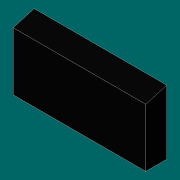
# Autodesk Inventor part: mirrorSuppourt
Saved by Autodesk Inventor 2016 (Build 200138000, 138)
## iProperties
Created: 2015-10-14
Part Number: mirrorSuppourt
Material: PC/ABS Plastic
Document SubType Name: Modeling
Designer: Sawaiz
Density: 0.357273 g/cm^3
Appearance: Smooth - Black
Author: Sawaiz
Autodesk Inventor part; units mm, degrees
ref_plane "YZ Plane" through (0, 0, 0) normal (1, 0, 0) x (0, 1, 0)
ref_plane "XZ Plane" through (0, 0, 0) normal (0, 1, 0) x (-1, 0, 0)
ref_plane "XY Plane" through (0, 0, 0) normal (0, 0, 1) x (1, 0, 0)
sketch "Sketch1" plane through (0, 0, 0) normal (0, 1, 0) x (-1, 0, 0)
  line L0 (0, 0) -> (77.9718, 23.8384)
  line L1 (78.376, 20.8249) -> (78.376, 0)
  line L2 (78.376, 0) -> (72.026, 0)
  line L3 (72.026, 0) -> (72.026, 18.8835)
  line L4 (0, 0) -> (50.5854, 0)
  line L5 (0, 0) -> (0.8771, -2.8689)
  line L6 (0.8771, -2.8689) -> (79.2531, 21.093)
  line L7 (79.2531, 21.093) -> (78.376, 23.9619)
  line L8 (78.376, 20.8249) -> (78.376, 23.9619)
  dimension "d0" = 6.35
  dimension "d1" = 17
  dimension "d2" = 78.376
  dimension "d5" = 3
  dimension "d6" = 3
  constraints: 18 end point, 4 perpendicular, 2 point on line, 2 vertical, 1 collinear, 1 horizontal, 1 parallel
  measures "d0" distance between parallel lines of L1 L3
  measures "d1" angle of L2 L0
  measures "d2" distance from line of L0.start L1
  measures "d5" distance between parallel lines of L0 L6
  measures "d6" distance of L6.end L7.end
extrude "Extrusion2" add sketch "Sketch1" along normal blind 40 contours L1 L2 L3 L6
equation "\"d0\" = acrylicThickness"
equation "\"d1\" = mirrorAngle"
equation "\"d2\" = -centerThickness + depth - aerogelThickness - fresnelThickness"
equation "\"d5\" = mirrorThickness"
equation "\"d6\" = mirrorThickness"
equation "\"d7\" = mirrorSuppourtWidth"
equation "\"acrylicThickness\" = 6.35"
equation "\"aerogelThickness\" = 20"
equation "\"depth\" = 100"
equation "\"mirrorAngle\" = 17deg"
equation "\"detectorWidth\" = 52"
equation "\"detectorHeight\" = 52"
equation "\"mirrorThickness\" = 3"
equation "\"fresnelThickness\" = 0.1"
equation "\"focalLength\" = 76.2"
equation "\"ior\" = 1.49"
equation "\"centerThickness\" = 1.524"
equation "\"fresnelAngle\" = 90deg"
equation "\"fresnelEffectiveDiameter\" = 76.2"
equation "\"mirrorSuppourtWidth\" = 40"
body "Solid2"
